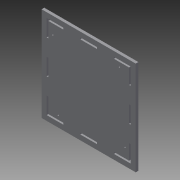
# Autodesk Inventor part: Bottom Panel
Saved by Autodesk Inventor 2015 SP1 (Build 190203100, 203)
## iProperties
Created: 2015-08-25
Part Number: Bottom Panel
Material: Generic
Document SubType Name: Modeling
Designer: Kartikye
Density: 1 g/cm^3
Appearance: Default
Author: Kartikye
Autodesk Inventor part; units mm, degrees
ref_plane "YZ Plane" through (0, 0, 0) normal (1, 0, 0) x (0, 1, 0)
ref_plane "XZ Plane" through (0, 0, 0) normal (0, 1, 0) x (-1, 0, 0)
ref_plane "XY Plane" through (0, 0, 0) normal (0, 0, 1) x (1, 0, 0)
sketch "Sketch1" plane through (0, 0, 0) normal (0, 1, 0) x (-1, 0, 0)
  line L0 (-28, 28) -> (28, 28)
  line L1 (28, 28) -> (28, -28)
  line L2 (28, -28) -> (-28, -28)
  line L3 (-28, -28) -> (-28, 28)
  line L4 (-28, 28) -> (28, -28) construction
  line L5 (28, 28) -> (-28, -28) construction
  point P0 (0, 0)
  dimension "d0" = 56
  dimension "d1" = 56
  constraints: 12 end point, 2 midpoint, 2 parallel, 1 horizontal, 1 perpendicular
  measures "d0" distance of L0.start L0.end
  measures "d1" distance of L0.end L1.end
extrude "Extrusion1" add sketch "Sketch1" along normal blind 1.6
sketch "Sketch2" plane through (0, 1.6, 0) normal (0, 1, 0) x (1, 0, 0)
  line L0 (25, -25) -> (-25, 25) construction
  line L1 (-25, -25) -> (25, 25) construction
  line L2 (-25, -25) -> (-25, -15)
  line L3 (-25, -15) -> (-24, -15)
  line L4 (-24, -15) -> (-24, -24)
  line L5 (-24, -24) -> (-15, -24)
  line L6 (-15, -24) -> (-15, -25)
  line L7 (15, -24) -> (15, -25)
  line L8 (-25, -25) -> (-15, -25)
  line L9 (-5, -25) -> (-5, -24)
  line L10 (-28, -28) -> (28, -28) projected
  line L11 (-25, 15) -> (-24, 15)
  line L12 (-25, -5) -> (-24, -5)
  line L13 (-24, -5) -> (-24, 5)
  line L14 (-24, 5) -> (-25, 5)
  line L15 (-25, -5) -> (-25, 5)
  line L16 (-28, 28) -> (-28, -28) projected
  line L17 (-5, 25) -> (-5, 24)
  line L18 (-5, 24) -> (5, 24)
  line L19 (5, 24) -> (5, 25)
  line L20 (25, 25) -> (15, 25)
  line L21 (15, 25) -> (15, 24)
  line L22 (15, 24) -> (24, 24)
  line L23 (24, 24) -> (24, 15)
  line L24 (24, 15) -> (25, 15)
  line L25 (-5, 25) -> (5, 25)
  line L26 (25, -5) -> (24, -5)
  line L27 (24, -5) -> (24, 5)
  line L28 (24, 5) -> (25, 5)
  line L29 (25, 5) -> (25, -5)
  line L30 (28, 28) -> (-28, 28) projected
  line L31 (25, 15) -> (25, 25)
  line L32 (15, -25) -> (25, -25)
  line L33 (25, -25) -> (25, -15)
  line L34 (25, -15) -> (24, -15)
  line L35 (24, -15) -> (24, -24)
  line L36 (15, -24) -> (24, -24)
  line L37 (-5, -25) -> (5, -25)
  line L38 (5, -25) -> (5, -24)
  line L39 (5, -24) -> (-5, -24)
  line L40 (-5, -24) -> (-5, -25)
  line L41 (-25, 15) -> (-25, 25)
  line L42 (-25, 25) -> (-15, 25)
  line L43 (-15, 25) -> (-15, 24)
  line L44 (-15, 24) -> (-24, 24)
  line L45 (-24, 15) -> (-24, 24)
  point P0 (0, 0)
  dimension "d4" = 50
  dimension "d5" = 50
  dimension "d6" = 10
  dimension "d7" = 1
  dimension "d8" = 9
  dimension "d9" = 9
  dimension "d16" = 10
  dimension "d17" = 10
  dimension "d18" = 1
  dimension "d21" = 1
  dimension "d22" = 10
  dimension "d23" = 3
  dimension "d24" = 10
  dimension "d25" = 1
  dimension "d27" = 10
  dimension "d28" = 10
  dimension "d29" = 1
  dimension "d30" = 9
  dimension "d31" = 9
  dimension "d32" = 1
  dimension "d33" = 10
  dimension "d34" = 1
  dimension "d35" = 10
  dimension "d36" = 3
  dimension "d37" = 10
  dimension "d38" = 10
  dimension "d39" = 10
  dimension "d40" = 10
  dimension "d41" = 10
  constraints: 86 end point, 12 perpendicular, 5 point on line, 5 vertical, 4 horizontal, 2 midpoint, 2 parallel
  measures "d4" distance of L0.start L1.start
  measures "d5" distance of L1.start L0.end
  measures "d6" distance of L1.start L2.end
  measures "d7" distance of L2.end L3.end
  measures "d8" distance of L3.end L4.end
  measures "d9" distance of L4.end L5.end
  measures "d16" distance between parallel lines of L9 L6
  measures "d17" distance of L0.end L11.start
  measures "d18" distance of L11.start L11.end
  measures "d21" distance of L12.start L12.end
  measures "d22" distance of L12.end L13.end
  measures "d23" distance between parallel lines of L15 L16
  measures "d24" distance between parallel lines of L12 L3
  measures "d25" distance of L17.start L17.end
  measures "d27" distance of L17.end L18.end
  measures "d28" distance of L1.end L20.end
  measures "d29" distance of L20.end L21.end
  measures "d30" distance of L21.end L22.end
  measures "d31" distance of L22.end L23.end
  measures "d32" distance of L26.start L26.end
  measures "d33" distance of L26.end L27.end
  measures "d34" distance of L27.end L28.end
  measures "d35" distance from line of L19 L20.end
  measures "d36" distance between parallel lines of L30 L25
  measures "d37" distance between parallel lines of L24 L28
  measures "d38" distance of L7.end L0.start
  measures "d39" distance of L0.start L33.end
  measures "d40" distance of L39.end L38.end
  measures "d41" distance of L0.end L42.end
extrude "Extrusion2" cut sketch "Sketch2" against normal blind 1.6
sketch "Sketch3" plane through (0, 1.6, 0) normal (0, 1, 0) x (1, 0, 0)
  circle A0 centre (-18.2, 21.5) radius 0.5
  circle A1 centre (21.5, 18.2) radius 0.5
  circle A2 centre (18.2, -21.5) radius 0.5
  circle A3 centre (-21.5, -18.2) radius 0.5
  line L0 (-25, -25) -> (-25, -15) projected
  line L1 (-15, -25) -> (-25, -25) projected
  line L2 (-25, 25) -> (-15, 25) projected
  line L3 (-25, 15) -> (-25, 25) projected
  line L4 (25, 25) -> (25, 15) projected
  line L5 (15, 25) -> (25, 25) projected
  line L6 (25, -15) -> (25, -25) projected
  line L7 (25, -25) -> (15, -25) projected
  point P0 (0, 0)
  dimension "d44" = 1
  dimension "d45" = 1
  dimension "d46" = 1
  dimension "d47" = 1
  dimension "d48" = 3.5
  dimension "d49" = 6.8
  dimension "d50" = 3.5
  dimension "d51" = 6.8
  dimension "d52" = 3.5
  dimension "d53" = 6.8
  dimension "d54" = 6.8
  dimension "d55" = 3.5
  constraints: 4 centre point
  measures "d44" diameter of A0
  measures "d45" diameter of A1
  measures "d46" diameter of A2
  measures "d47" diameter of A3
  measures "d48" distance from line of L0 A3.centre
  measures "d49" distance from line of L1 A3.centre
  measures "d50" distance from line of L2 A0.centre
  measures "d51" distance from line of A0.centre L3
  measures "d52" distance from line of A1.centre L4
  measures "d53" distance from line of A1.centre L5
  measures "d54" distance from line of A2.centre L6
  measures "d55" distance from line of L7 A2.centre
extrude "Extrusion3" cut sketch "Sketch3" against normal blind 1.6
body "Solid1"
